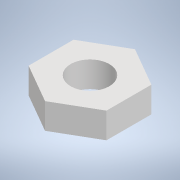
# Autodesk Inventor part: Nut
Saved by Autodesk Inventor 2021 (Build 250183000, 183)
## iProperties
Created: 2021-08-04
Part Number: Nut
Material: Generic
Document SubType Name: Modeling
Designer: techv
Density: 1 g/cm^3
Appearance: Default
Author: techv
Autodesk Inventor part; units mm, degrees
ref_plane "YZ Plane" through (0, 0, 0) normal (1, 0, 0) x (0, 1, 0)
ref_plane "XZ Plane" through (0, 0, 0) normal (0, 1, 0) x (-1, 0, 0)
ref_plane "XY Plane" through (0, 0, 0) normal (0, 0, 1) x (1, 0, 0)
sketch "Sketch1" plane through (0, 0, 0) normal (0, 1, 0) x (-1, 0, 0)
  circle A0 centre (2.2281, 5.8523) radius 1.5 projected
  circle A1 centre (2.2281, 5.8523) radius 3.5
  line L0 (2.2281, 2.3523) -> (-0.803, 4.1023)
  line L1 (-0.803, 4.1023) -> (-0.803, 7.6023)
  line L2 (-0.803, 7.6023) -> (2.2281, 9.3523)
  line L3 (2.2281, 9.3523) -> (5.2592, 7.6023)
  line L4 (5.2592, 7.6023) -> (5.2592, 4.1023)
  line L5 (5.2592, 4.1023) -> (2.2281, 2.3523)
  point P0 (0, 0)
  dimension "d0" = 7
  constraints: 12 end point, 2 coincident, 1 vertical alignment, 15 other
extrude "Extrusion1" add sketch "Sketch1" against normal blind 2 contours L4 L5 L0 L1 L2 L3
thread "Thread1" size "M3x0.5" class "6H" standard "ANSI Metric M Profile" full length
sketch "Sketch2" plane through (0, -2, 0) normal (0, -1, 0) x (1, 0, 0)
  line L0 (-5.2592, 7.6023) -> (-5.2592, 4.1023) projected
  line L1 (-5.2592, 4.1023) -> (-2.2281, 2.3523) projected
  line L2 (-2.2281, 2.3523) -> (0.803, 4.1023) projected
  line L3 (0.803, 4.1023) -> (0.803, 7.6023) projected
  line L4 (0.803, 7.6023) -> (-2.2281, 9.3523) projected
  line L5 (-2.2281, 9.3523) -> (-5.2592, 7.6023) projected
  circle A0 centre (-2.2281, 5.8523) radius 1.5 projected
  line L6 (-7.2281, 0.8523) -> (2.7719, 0.8523)
  line L7 (2.7719, 0.8523) -> (2.7719, 10.8523)
  line L8 (2.7719, 10.8523) -> (-7.2281, 10.8523)
  line L9 (-7.2281, 10.8523) -> (-7.2281, 0.8523)
  line L10 (-7.2281, 0.8523) -> (2.7719, 10.8523) construction
  line L11 (2.7719, 0.8523) -> (-7.2281, 10.8523) construction
  point P0 (0, 0)
  dimension "d5" = 10
  dimension "d6" = 10
  constraints: 12 end point, 2 midpoint, 2 parallel, 1 horizontal, 1 perpendicular
  measures "d5" distance of L8.end L7.end
  measures "d6" distance of L7.end L6.end
extrude "Extrusion2" add sketch "Sketch2" against normal blind 2 contours L9 L8 L7 L6
sketch "Sketch3" plane through (0, 0, 0) normal (0, 1, 0) x (1, 0, 0)
  line L0 (2.7719, -10.8523) -> (2.7719, -0.8523) projected
  line L1 (2.7719, -0.8523) -> (-7.2281, -0.8523) projected
  line L2 (-7.2281, -0.8523) -> (-7.2281, -10.8523) projected
  line L3 (-7.2281, -10.8523) -> (2.7719, -10.8523) projected
  circle A0 centre (-2.2281, -5.8523) radius 1.5 projected
  line L4 (-8.7281, 0.6477) -> (4.2719, 0.6477)
  line L5 (4.2719, 0.6477) -> (4.2719, -12.3523)
  line L6 (4.2719, -12.3523) -> (-8.7281, -12.3523)
  line L7 (-8.7281, -12.3523) -> (-8.7281, 0.6477)
  line L8 (-8.7281, 0.6477) -> (4.2719, -12.3523) construction
  line L9 (4.2719, 0.6477) -> (-8.7281, -12.3523) construction
  point P0 (0, 0)
  dimension "d9" = 10
  dimension "d10" = 13
  dimension "d11" = 13
  constraints: 12 end point, 2 midpoint, 2 parallel, 1 horizontal, 1 perpendicular
  measures "d9" distance between parallel lines of L3 L1
  measures "d10" distance of L5.end L6.end
  measures "d11" distance of L4.end L5.end
extrude "Extrusion3" add sketch "Sketch3" along normal blind 100 and the other way blind 3 contours L4 L5 L6 L7
sketch "Sketch4" plane through (0, 100, 0) normal (0, 1, 0) x (1, 0, 0)
  line L0 (-8.7281, -12.3523) -> (4.2719, -12.3523) projected
  line L1 (4.2719, -12.3523) -> (4.2719, 0.6477) projected
  line L2 (4.2719, 0.6477) -> (-8.7281, 0.6477) projected
  line L3 (-8.7281, 0.6477) -> (-8.7281, -12.3523) projected
  line L4 (2.7719, -10.8523) -> (-7.2281, -10.8523) projected
  line L5 (-7.2281, -10.8523) -> (-7.2281, -0.8523) projected
  line L6 (-7.2281, -0.8523) -> (2.7719, -0.8523) projected
  line L7 (2.7719, -0.8523) -> (2.7719, -10.8523) projected
  point P0 (0, 0)
extrude "Extrusion4" add sketch "Sketch4" against normal blind 3 contours L4 L5 L6 L7
body "Solid1"
